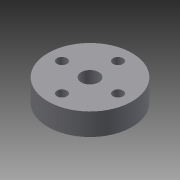
# Autodesk Inventor part: Motor_Hub_Polulu
Saved by Autodesk Inventor 2015 SP1 (Build 190203100, 203)
## iProperties
Created: 2016-04-07
Part Number: Motor_Hub_Polulu
Material: Generic
Document SubType Name: Modeling
Designer: Ethan
Density: 1 g/cm^3
Appearance: Default
Author: Ethan
Autodesk Inventor part; units mm, degrees
ref_plane "YZ Plane" through (0, 0, 0) normal (1, 0, 0) x (0, 1, 0)
ref_plane "XZ Plane" through (0, 0, 0) normal (0, 1, 0) x (-1, 0, 0)
ref_plane "XY Plane" through (0, 0, 0) normal (0, 0, 1) x (1, 0, 0)
sketch "Sketch1" plane through (0, 0, 0) normal (0, 1, 0) x (-1, 0, 0)
  circle A0 centre (0, 0) radius 9.5
  circle A1 centre (0, 0) radius 2
  circle A2 centre (-6.35, 0) radius 1.1303
  circle A3 centre (0, -6.35) radius 1.1303
  circle A4 centre (6.35, 0) radius 1.1303
  circle A5 centre (0, 6.35) radius 1.1303
  dimension "d0" = 19
  dimension "d1" = 4
  dimension "d2" = 6.35
  dimension "d3" = 2.2606
  dimension "d6" = 360
  constraints: 6 centre point, 2 coincident, 9 other
  measures "d0" diameter of A0
  measures "d1" diameter of A1
  measures "d2" distance of point (0, 0) A2.centre
  measures "d3" diameter of A2
extrude "Extrusion1" add sketch "Sketch1" along normal blind 5
body "Solid1"
